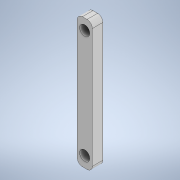
# Autodesk Inventor part: hank - linkage
Saved by Autodesk Inventor 2022 (Build 260153000, 153)
## iProperties
Created: 2022-01-19
Part Number: hank - linkage
Material: Generic
Document SubType Name: Modeling
Designer: chris
Density: 1 g/cm^3
Appearance: Default
Author: chris
Autodesk Inventor part; units mm, degrees
ref_plane "YZ Plane" through (0, 0, 0) normal (1, 0, 0) x (0, 1, 0)
ref_plane "XZ Plane" through (0, 0, 0) normal (0, 1, 0) x (-1, 0, 0)
ref_plane "XY Plane" through (0, 0, 0) normal (0, 0, 1) x (1, 0, 0)
sketch "Sketch1" plane through (0, 0, 0) normal (0, 0, 1) x (1, 0, 0)
  line L0 (-2.286, -3.4798) -> (2.286, -3.4798)
  line L1 (-2.286, -3.4798) -> (-2.286, 33.3502)
  line L2 (-2.286, 33.3502) -> (2.286, 33.3502)
  line L3 (2.286, 33.3502) -> (2.286, -3.4798)
  line L4 (2.286, 14.9352) -> (-2.286, 14.9352)
  line L5 (0, 33.3502) -> (0, 31.242)
  circle A0 centre (0, 31.242) radius 1.524
  circle A1 centre (0, -1.3716) radius 1.524
  line L6 (0, -3.4798) -> (0, -4.6228)
  line L7 (0, -4.6228) -> (2.286, -4.6228)
  line L8 (2.286, -4.6228) -> (2.286, -3.4798)
  line L9 (-2.286, -3.4798) -> (-2.286, -4.6228)
  line L10 (-2.286, -4.6228) -> (0, -4.6228)
  line L11 (0, 34.4932) -> (2.286, 34.4932)
  line L12 (2.286, 34.4932) -> (2.286, 33.3502)
  line L13 (-2.286, 33.3502) -> (-2.286, 34.4932)
  line L14 (-2.286, 34.4932) -> (0, 34.4932)
  point P0 (0, 0)
  dimension "d0" = 4.572
  dimension "d1" = 36.83
  dimension "d2" = 2.1082
  dimension "d3" = 3.048
  dimension "d7" = 1.143
  constraints: 30 end point, 4 midpoint, 4 perpendicular, 4 symmetric about line, 3 vertical, 2 centre point, 2 horizontal, 2 point on line, 1 coincident, 1 parallel, 1 vertical alignment, 1 other
  measures "d0" distance of L0.start L0.end
  measures "d1" distance of L0.start L1.end
  measures "d2" distance of L5.start L5.end
  measures "d3" diameter of A0
  measures "d7" distance of L6.start L6.end
extrude "Extrusion1" add sketch "Sketch1" along normal blind 3.175
fillet "Fillet2" radius 1.5875 4 edges at (2.286, 34.4932, 1.5875) (-2.286, 34.4932, 1.5875) (-2.286, -4.6228, 1.5875) (2.286, -4.6228, 1.5875)
body "Solid1"
